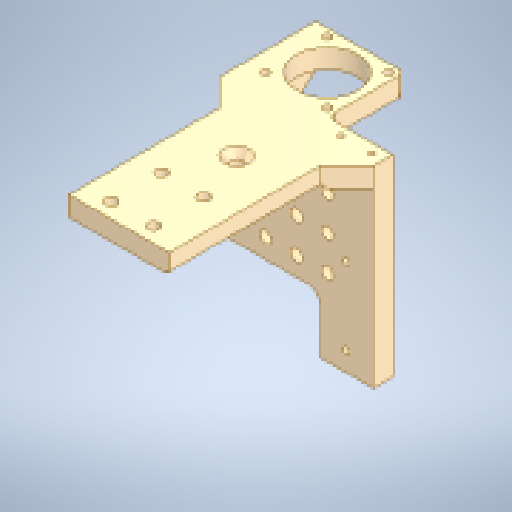
# Autodesk Inventor part: Motor_holder_R
Saved by Autodesk Inventor 2024.1 (Build 281209000, 209)
## iProperties
Created: 2023-09-16
Part Number: Motor_holder_R
Material: ABS Plastic
Document SubType Name: Modeling
Designer: l1534
Density: 1.06 g/cm^3
Appearance: Smooth - Off-White
Author: l1534
Autodesk Inventor part; units mm, degrees
ref_plane "YZ Plane" through (0, 0, 0) normal (1, 0, 0) x (0, 1, 0)
ref_plane "XZ Plane" through (0, 0, 0) normal (0, 1, 0) x (-1, 0, 0)
ref_plane "XY Plane" through (0, 0, 0) normal (0, 0, 1) x (1, 0, 0)
sketch "Sketch1" plane through (0, 0, 0) normal (0, 0, 1) x (1, 0, 0)
  line L0 (-10.4918, 19.8361) -> (-50.4918, 19.8361)
  line L1 (-50.4918, 19.8361) -> (-50.4918, -15.1639)
  line L2 (-50.4918, -15.1639) -> (-10.4918, -15.1639)
  line L3 (-10.4918, -15.1639) -> (-10.4918, 19.8361)
  point P0 (0, 0)
  dimension "d0" = 40
  dimension "d1" = 35
  constraints: 8 end point, 2 parallel, 1 horizontal, 1 perpendicular
  measures "d0" distance of L0.start L0.end
  measures "d1" distance of L0.end L1.end
extrude "Extrusion1" add sketch "Sketch1" along normal blind 5
sketch "Sketch2" plane through (0, 0, 0) normal (0, 0, -1) x (-1, 0, 0)
  line L0 (50.4918, 19.8361) -> (50.4918, -15.1639) projected
  line L1 (50.4918, 19.8361) -> (27.4918, 19.8361)
  line L2 (27.4918, 19.8361) -> (27.4918, 14.8361)
  line L3 (27.4918, 14.8361) -> (50.4918, 14.8361)
  line L4 (50.4918, 14.8361) -> (50.4918, 19.8361)
  point P0 (0, 0)
  point P1 (50.4918, 14.8361)
  dimension "d4" = 23
  dimension "d5" = 5
  constraints: 8 end point, 2 parallel, 1 horizontal, 1 perpendicular
  measures "d4" distance of L2.end L3.end
  measures "d5" distance of L1.end L2.end
extrude "Extrusion2" add sketch "Sketch2" along normal blind 20
sketch "Sketch3" plane through (0, 0, 0) normal (0, 0, -1) x (-1, 0, 0)
  line L0 (27.4918, 14.8361) -> (50.4918, 14.8361) projected
  line L1 (50.4918, 19.8361) -> (50.4918, -15.1639) projected
  line L2 (50.4918, 15.8361) -> (47.4918, 15.8361)
  line L3 (47.4918, 15.8361) -> (47.4918, -4.1639)
  line L4 (47.4918, -4.1639) -> (50.4918, -4.1639)
  line L5 (50.4918, -4.1639) -> (50.4918, 15.8361)
  point P0 (0, 0)
  point P1 (47.4918, 14.8361)
  dimension "d8" = 20
  dimension "d9" = 3
  constraints: 8 end point, 2 parallel, 1 horizontal, 1 perpendicular, 1 point on line
  measures "d8" distance of L2.end L3.end
  measures "d9" distance of L3.end L4.end
extrude "Extrusion3" add sketch "Sketch3" along normal blind 20 contours L0 L1 L4 L3
sketch "Sketch4" plane through (-27.4918, 14.8361, -20) normal (0, -1, 0) x (1, 0, 0)
  circle A0 centre (-10, 10) radius 8
  line L0 (0, 0) -> (-20, 0) projected
  line L1 (0, 20) -> (0, 0) projected
  circle A1 centre (-2, 2) radius 1
  circle A2 centre (-18, 2) radius 1
  circle A3 centre (-18, 18) radius 1
  circle A4 centre (-2, 18) radius 1
  point P0 (27.4918, 20)
  dimension "d12" = 16
  dimension "d13" = 10
  dimension "d14" = 10
  dimension "d15" = 2
  dimension "d16" = 2
  dimension "d17" = 2
  dimension "d18" = 2
  dimension "d19" = 8
  dimension "d20" = 8
  dimension "d21" = 8
  dimension "d22" = 8
  dimension "d23" = 8
  dimension "d24" = 8
  dimension "d25" = 8
  dimension "d26" = 8
  constraints: 5 centre point
  measures "d12" diameter of A0
  measures "d13" distance from line of L0 A0.centre
  measures "d14" distance from line of L1 A0.centre
  measures "d15" diameter of A1
  measures "d16" diameter of A2
  measures "d17" diameter of A3
  measures "d18" diameter of A4
  measures "d19" horizontal distance of A0.centre A1.centre
  measures "d20" horizontal distance of A0.centre A1.centre
  measures "d21" horizontal distance of A0.centre A2.centre
  measures "d22" horizontal distance of A0.centre A2.centre
  measures "d23" horizontal distance of A0.centre A3.centre
  measures "d24" horizontal distance of A0.centre A3.centre
  measures "d25" horizontal distance of A0.centre A4.centre
  measures "d26" horizontal distance of A0.centre A4.centre
extrude "Extrusion4" cut sketch "Sketch4" against normal through all
fillet "Fillet1" radius 1.5 1 edges at (-27.4918, 17.3361, -20)
sketch "Sketch5" plane through (-47.4918, -4.1639, 0) normal (1, 0, 0) x (0, 0, -1)
  line L0 (20, 19) -> (20, 0) projected
  line L1 (0, 0) -> (20, 0) projected
  line L2 (20, 19) -> (0, 0)
  line L3 (0, 0) -> (20, 0)
  line L4 (20, 0) -> (20, 19)
  point P0 (0, 4.1639)
  constraints: 6 end point, 1 horizontal, 1 perpendicular, 1 point on line
extrude "Extrusion5" cut sketch "Sketch5" against normal through all
fillet "Fillet2" radius 5 1 edges at (-48.9918, -4.1639, 0)
fillet "Fillet4" radius 2 1 edges at (-47.4918, 5.3361, 0)
sketch "Sketch6" plane through (0, 0, 5) normal (0, 0, 1) x (1, 0, 0)
  line L0 (-10.4918, 19.8361) -> (-50.4918, 19.8361) projected
  line L1 (-17.4918, 19.8361) -> (-43.4918, 19.8361)
  line L2 (-43.4918, 19.8361) -> (-43.4918, 14.8361)
  line L3 (-43.4918, 14.8361) -> (-17.4918, 14.8361)
  line L4 (-17.4918, 14.8361) -> (-17.4918, 19.8361)
  line L5 (-10.4918, -15.1639) -> (-10.4918, 19.8361) projected
  line L6 (-50.4918, 19.8361) -> (-50.4918, -15.1639) projected
  point P0 (0, 0)
  dimension "d39" = 5
  dimension "d40" = 7
  dimension "d41" = 7
  constraints: 8 end point, 2 parallel, 1 horizontal, 1 perpendicular, 1 point on line
  measures "d39" distance of L3.end L1.start
  measures "d40" distance between parallel lines of L5 L4
  measures "d41" distance between parallel lines of L6 L2
extrude "Extrusion6" add sketch "Sketch6" along normal blind 46
chamfer "Chamfer2" distance 7 angle 45 2 edges at (-17.4918, 17.3361, 5) (-43.4918, 17.3361, 5)
sketch "Sketch7" plane through (-43.4918, 14.8361, 51) normal (0, -1, 0) x (1, 0, 0)
  circle A0 centre (13, -30.5) radius 1.5
  line L0 (-7, -46) -> (33, -46) projected
  line L1 (26, -39) -> (26, 0) projected
  point P0 (43.4918, -51)
  dimension "d47" = 3
  dimension "d48" = 15.5
  dimension "d49" = 13
  constraints: 1 centre point
  measures "d47" diameter of A0
  measures "d48" distance from line of L0 A0.centre
  measures "d49" distance from line of L1 A0.centre
extrude "Extrusion7" cut sketch "Sketch7" against normal through all
chamfer "Chamfer3" distance 1.8 angle 45 1 edges at (-31.9918, 19.8361, 20.5)
sketch "Sketch8" plane through (-27.4918, 19.8361, 0) normal (0, 1, 0) x (1, 0, 0)
  circle A0 centre (14, -2.5) radius 0.8
  circle A1 centre (6, -2.5) radius 0.8
  line L0 (17, 0) -> (0, 0) projected
  line L1 (17, 0) -> (17, -5) projected
  point P0 (27.4918, 0)
  dimension "d55" = 1.6
  dimension "d56" = 1.6
  dimension "d57" = 2.5
  dimension "d58" = 2.5
  dimension "d59" = 3
  dimension "d60" = 8
  constraints: 2 centre point
  measures "d55" diameter of A0
  measures "d56" diameter of A1
  measures "d57" distance from line of L0 A0.centre
  measures "d58" distance from line of L0 A1.centre
  measures "d59" distance from line of L1 A0.centre
  measures "d60" distance of A0.centre A1.centre
extrude "Extrusion8" cut sketch "Sketch8" against normal blind 10
chamfer "Chamfer4" distance 0.8 angle 45 2 edges at (-14.2918, 9.8361, 2.5) (-22.2918, 9.8361, 2.5)
fillet "Fillet5" radius 1 2 edges at (-14.2918, 10.6356, 2.5) (-22.2918, 10.6356, 2.5)
sketch "Sketch9" plane through (-50.4918, -15.1639, 0) normal (0, -1, 0) x (1, 0, 0)
  line L0 (40, 0) -> (40, 5) projected
  line L1 (40, 0) -> (23, 0) projected
  line L2 (40, 5) -> (26, 5)
  line L3 (26, 5) -> (26, 0)
  line L4 (26, 0) -> (40, 0)
  line L5 (40, 0) -> (40, 5)
  point P0 (50.4918, 0)
  dimension "d67" = 14
  constraints: 8 end point, 2 parallel, 1 horizontal, 1 perpendicular, 1 point on line
  measures "d67" distance between parallel lines of L0 L3
extrude "Extrusion9" add sketch "Sketch9" along normal blind 15
sketch "Sketch10" plane through (0, 0, 0) normal (0, 0, -1) x (-1, 0, 0)
  circle A0 centre (17.4918, -25.1639) radius 0.8
  line L0 (10.4918, 19.8361) -> (10.4918, -30.1639) projected
  line L1 (24.4918, -30.1639) -> (10.4918, -30.1639) projected
  circle A1 centre (17.4918, -5.1639) radius 0.8
  circle A2 centre (17.4918, 14.8361) radius 0.8
  point P0 (0, 0)
  dimension "d70" = 1.6
  dimension "d71" = 7
  dimension "d72" = 5
  dimension "d75" = 20
  constraints: 3 centre point, 1 vertical, 4 other
  measures "d70" diameter of A0
  measures "d71" distance from line of L0 A0.centre
  measures "d72" distance from line of L1 A0.centre
  measures "d75" distance of A0.centre A1.centre
extrude "Extrusion10" cut sketch "Sketch10" against normal through all
fillet "Fillet6" radius 3 2 edges at (-50.4918, -15.1639, 2.5) (-24.4918, -15.1639, 2.5)
sketch "Sketch11" plane through (0, 0, 0) normal (0, 0, -1) x (-1, 0, 0)
  circle A0 centre (38.4918, -10.1639) radius 1.5
  circle A1 centre (30.4918, -10.1639) radius 1.5
  circle A2 centre (30.4918, -1.1639) radius 1.5
  circle A3 centre (38.4918, -1.1639) radius 1.5
  circle A4 centre (38.4918, 7.8361) radius 1.5
  circle A5 centre (30.4918, 7.8361) radius 1.5
  line L0 (47.4918, -15.1639) -> (27.4918, -15.1639) projected
  line L1 (50.4918, -6.3105) -> (50.4918, -12.1639) projected
  circle A6 centre (22.4918, -10.1639) radius 1.5
  circle A7 centre (22.4918, -1.1639) radius 1.5
  circle A8 centre (22.4918, 7.8361) radius 1.5
  point P0 (0, 0)
  point P1 (37.4918, -15.1639)
  dimension "d89" = 3
  dimension "d90" = 3
  dimension "d91" = 3
  dimension "d92" = 3
  dimension "d93" = 3
  dimension "d94" = 3
  dimension "d95" = 5
  dimension "d96" = 5
  dimension "d97" = 8
  dimension "d98" = 12
  dimension "d99" = 12
  dimension "d100" = 12
  dimension "d101" = 9
  dimension "d102" = 9
  dimension "d103" = 9
  dimension "d104" = 8
  dimension "d105" = 9
  dimension "d106" = 8
  dimension "d109" = 8
  dimension "d110" = 3
  dimension "d111" = 5
  dimension "d112" = 9
  dimension "d113" = 9
  dimension "d114" = 3
  dimension "d115" = 3
  dimension "d116" = 8
  dimension "d117" = 8
  constraints: 9 centre point, 1 midpoint
  measures "d89" diameter of A5
  measures "d90" diameter of A4
  measures "d91" diameter of A3
  measures "d92" diameter of A2
  measures "d93" diameter of A1
  measures "d94" diameter of A0
  measures "d95" vertical distance of point (37.492, -15.164) A1.centre
  measures "d96" distance from line of L0 A0.centre
  measures "d97" distance of A0.centre A1.centre
  measures "d98" distance from line of L1 A0.centre
  measures "d99" distance from line of L1 A3.centre
  measures "d100" distance from line of L1 A4.centre
  measures "d101" distance of A0.centre A3.centre
  measures "d102" distance of A4.centre A3.centre
  measures "d103" distance of A1.centre A2.centre
  measures "d104" distance of A3.centre A2.centre
  measures "d105" distance of A2.centre A5.centre
  measures "d106" distance of A4.centre A5.centre
  measures "d109" distance of A1.centre A6.centre
  measures "d110" diameter of A6
  measures "d111" distance from line of L0 A6.centre
  measures "d112" distance of A6.centre A7.centre
  measures "d113" distance of A8.centre A7.centre
  measures "d114" diameter of A8
  measures "d115" diameter of A7
  measures "d116" distance of A5.centre A8.centre
  measures "d117" distance of A2.centre A7.centre
extrude "Extrusion11" cut sketch "Sketch11" against normal through all
chamfer "Chamfer7" distance 1.9 angle 45 9 edges at (-20.9918, 7.8361, 0) (-20.9918, -1.1639, 0) (-20.9918, -10.1639, 0) (-28.9918, -10.1639, 0) (-28.9918, -1.1639, 0) (-28.9918, 7.8361, 0) (-36.9918, 7.8361, 0) (-36.9918, -1.1639, 0) (-36.9918, -10.1639, 0)
sketch "Sketch12" plane through (-27.4918, 19.8361, 0) normal (0, 1, 0) x (1, 0, 0)
  circle A0 centre (2, -34) radius 1.5
  circle A1 centre (2, -47) radius 1.5
  circle A2 centre (-9, -34) radius 1.5
  circle A3 centre (-9, -47) radius 1.5
  line L0 (10, -51) -> (-16, -51) projected
  line L1 (10, -12) -> (10, -51) projected
  line L2 (-16, -12) -> (-16, -51) projected
  point P0 (27.4918, 0)
  dimension "d121" = 3
  dimension "d122" = 3
  dimension "d123" = 3
  dimension "d124" = 3
  dimension "d125" = 17
  dimension "d126" = 17
  dimension "d127" = 8
  dimension "d128" = 8
  dimension "d129" = 7
  dimension "d130" = 7
  dimension "d131" = 4
  dimension "d132" = 4
  constraints: 4 centre point
  measures "d121" diameter of A0
  measures "d122" diameter of A2
  measures "d123" diameter of A1
  measures "d124" diameter of A3
  measures "d125" distance from line of L0 A2.centre
  measures "d126" distance from line of L0 A0.centre
  measures "d127" distance from line of L1 A1.centre
  measures "d128" distance from line of L1 A0.centre
  measures "d129" distance from line of L2 A2.centre
  measures "d130" distance from line of L2 A3.centre
  measures "d131" distance from line of L0 A3.centre
  measures "d132" distance from line of L0 A1.centre
extrude "Extrusion12" cut sketch "Sketch12" against normal through all
fillet "Fillet7" radius 3 1 edges at (-27.4918, 17.3361, 0)
body "Solid1"
